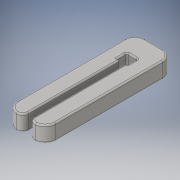
# Autodesk Inventor part: BaseClip
Saved by Autodesk Inventor 2016 (Build 200138000, 138)
## iProperties
Created: 2016-03-05
Part Number: BaseClip
Material: Generic
Document SubType Name: Modeling
Designer: yash
Density: 1 g/cm^3
Appearance: Default
Author: yash
Autodesk Inventor part; units mm, degrees
ref_plane "YZ Plane" through (0, 0, 0) normal (1, 0, 0) x (0, 1, 0)
ref_plane "XZ Plane" through (0, 0, 0) normal (0, 1, 0) x (-1, 0, 0)
ref_plane "XY Plane" through (0, 0, 0) normal (0, 0, 1) x (1, 0, 0)
sketch "Sketch1" plane through (0, 0, 0) normal (0, 1, 0) x (-1, 0, 0)
  line L0 (0, 0) -> (-4.7625, 0)
  line L1 (-4.7625, 0) -> (-4.7625, -28.575)
  line L2 (0, -1.7454) -> (0, 0)
  line L3 (-4.7625, -31.75) -> (-6.35, -31.75)
  line L4 (-11.43, -1.7454) -> (-11.43, -38.1)
  line L5 (-11.43, -38.1) -> (0, -38.1)
  line L6 (0, -38.1) -> (0, -1.7454)
  line L7 (-6.6675, -28.575) -> (-6.6675, 0)
  line L8 (-6.6675, 0) -> (-11.43, 0)
  line L9 (-11.43, 0) -> (-11.43, -1.7454)
  line L10 (-3.9688, -31.75) -> (-7.1437, -31.75)
  line L11 (-7.1437, -31.75) -> (-7.1438, -28.575)
  line L12 (-3.9688, -28.575) -> (-3.9688, -31.75)
  line L13 (-7.1438, -28.575) -> (-6.6675, -28.575)
  line L14 (-4.7625, -28.575) -> (-3.9688, -28.575)
  point P0 (-5.5563, -31.75)
  point P1 (-5.5562, -31.75)
  dimension "d12" = 38.1
  dimension "d13" = 6.35
  dimension "d14" = 4.7625
  dimension "d20" = 3.175
  dimension "d21" = 3.175
  dimension "d22" = 1.905
  dimension "d23" = 3.9688
  dimension "d24" = 31.75
  dimension "d25" = 1.7454
  dimension "d26" = 4.7625
  dimension "d27" = 28.575
  constraints: 30 end point, 7 parallel, 3 horizontal, 3 perpendicular, 2 equal length, 2 midpoint, 1 coincident, 1 collinear
  measures "d12" distance between parallel lines of L8 L5
  measures "d13" distance between parallel lines of L5 L3
  measures "d14" distance between parallel lines of L4 L7
  measures "d20" distance of L10.start L10.end
  measures "d21" distance of L10.end L11.end
  measures "d22" distance between parallel lines of L1 L7
  measures "d23" distance between parallel lines of L12 L2
  measures "d24" distance between parallel lines of L3 L0
  measures "d25" distance from line of L2.start L0
  measures "d26" distance from line of L3.start L2
  measures "d27" distance between parallel lines of L14 L0
extrude "Extrusion1" add sketch "Sketch1" along normal blind 4.7625
fillet "Fillet1" radius 3.175 4 edges at (0, 2.3813, -38.1) (11.43, 2.3813, -38.1) (0, 2.3813, 0) (11.43, 2.3813, 0)
fillet "Fillet2" radius 1.7272 2 edges at (6.6675, 2.3813, 0) (4.7625, 2.3813, 0)
fillet "Fillet3" radius 0.4318 22 edges at (10.5001, 4.7625, -37.1701) (5.715, 4.7625, -38.1) (0.9299, 4.7625, -37.1701) (0, 4.7625, -19.05) (0.8169, 4.7625, -1.0489) (4.1962, 4.7625, -0.4551) (4.7625, 4.7625, -15.1545) (10.6131, 4.7625, -1.0489) (7.2338, 4.7625, -0.4551) (6.6675, 4.7625, -15.1545) (11.43, 4.7625, -19.05) (10.5001, 0, -37.1701) (5.715, 0, -38.1) (0.9299, 0, -37.1701) (0, 0, -19.05) (0.8169, 0, -1.0489) (4.1962, 0, -0.4551) (4.7625, 0, -15.1545) (10.6131, 0, -1.0489) (7.2338, 0, -0.4551) (6.6675, 0, -15.1545) (11.43, 0, -19.05)
fillet "Fillet4" radius 0.4318 8 edges at (3.9688, 4.7625, -30.1625) (7.1438, 4.7625, -30.1625) (5.5563, 4.7625, -31.75) (3.9688, 0, -30.1625) (5.5563, 0, -31.75) (7.1438, 0, -30.1625) (7.1437, 2.3813, -31.75) (3.9688, 2.3813, -31.75)
body "Solid1"
